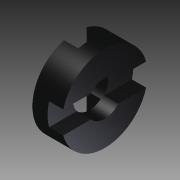
# Autodesk Inventor part: MCOC_spacer17
Saved by Autodesk Inventor 2011 SP1 (Build 150282100, 282)
## iProperties
Created: 2015-02-02
Part Number: MCOC_spacer17
Catalog Web Link: www.cadenas.de
Description: MCOC  Spacer-Couplings - Spacers
Vendor: MISUMI
Document SubType Name: Modeling
Designer: PARTuser1
Manufacturer: MISUMI
Mass: 0.915493 g
Surface Area: 8.84942 cm^2
Volume: 0.915493 cm^3
Density: 1 g/cm^3
Category: PARTsolutions
Company: MISUMI
Title: MCOC_spacer17
Author: Cadenas PARTsolutions
Comments: Couplings - Spacers
PSOL_IDENT_0: {\\10.0.0.236\data_v8\23d-libs\misumi\metric\50_couplings\parts\mcoc_spacer.prj},174 {VTYP=3D},{NB=M
PSOL_IDENT_1: COC_spacer17},{LINA=MCOC_spacer17},{NN=MCOC  Spacer},{DATE=13.11.2014 06:59:38},{GEOMDATE=22.08.2008
PSOL_IDENT_2: 00:00:00},{VERSION=},{LINEID=60},{LINESUBID=-1},{WBVAR=}  {NB=MCOC_spacer17},{LINA=MCOC_spacer17},{
PSOL_IDENT_3: KT=DUMMY},{PN=MCOC_spacer17},{MAT=Carbon Reinforced Resin},{TYPE=MCOC_spacer},{NO=17},{D1=17.5},{T=6
PSOL_IDENT_4: .0},{DD3=7.2},{W=4.6},{G=2.9},{Z=4.440},{Z1=1.200}
SUPPLIER: MISUMI
ARTICLENO: MCOC_spacer17
BOMINFO: MCOC_spacer17
CREATOR: CADENAS GmbH
Autodesk Inventor part; units mm, degrees
sketch "Sketch_1" plane through (0, 0, 0) normal (0, 0, 1) x (1, 0, 0)
  line L0 (6, 0) -> (0, 0)
  line L1 (0, 8.75) -> (0, 3.6)
  line L2 (0, 3.6) -> (6, 3.6)
  line L3 (6, 3.6) -> (6, 8.75)
  line L4 (6, 8.75) -> (0, 8.75)
  constraints: 10 end point
revolve "Revolution1" add sketch "Sketch_1" angle 360 about axis through (6, 0, 0) along (1, 0, 0)
sketch "Sketch_2" plane through (0, 0, 0) normal (0, 0, 1) x (1, 0, 0)
  line L0 (0, -2.3) -> (2.9, -2.3)
  line L1 (2.9, -2.3) -> (2.9, 2.3)
  line L2 (2.9, 2.3) -> (0, 2.3)
  line L3 (0, 2.3) -> (0, -2.3)
  constraints: 8 end point
extrude "Extrusion1" cut sketch "Sketch_2" along normal mid plane 17.5
sketch "Sketch_3" plane through (0, 0, 0) normal (0, 1, 0) x (-1, 0, 0)
  line L0 (-3.1, -2.3) -> (-3.1, 2.3)
  line L1 (-3.1, 2.3) -> (-6, 2.3)
  line L2 (-6, 2.3) -> (-6, -2.3)
  line L3 (-6, -2.3) -> (-3.1, -2.3)
  constraints: 8 end point
extrude "Extrusion2" cut sketch "Sketch_3" along normal mid plane 17.5
ref_plane "C_XY" through (3, 0, 0) normal (1, 0, 0) x (0, 0, -1)
ref_plane "C_YZ" through (3, 0, 0) normal (0, 0, -1) x (0, 1, 0)
ref_plane "C_ZX" through (3, 0, 0) normal (0, 1, 0) x (1, 0, 0)
body "Solid1"
